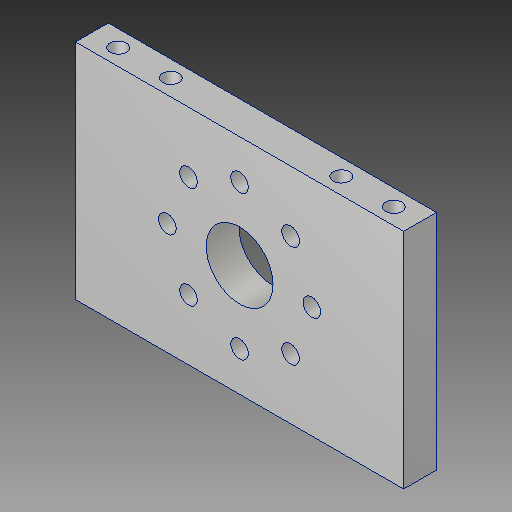
# Autodesk Inventor part: Box_Top
Saved by Autodesk Inventor 2019 (Build 230136000, 136)
## iProperties
Created: 2021-07-28
Part Number: Box_Top
Material: 알루미늄 6061
Document SubType Name: Modeling
Designer: user
Density: 2.7 g/cm^3
Appearance: 알루미늄 - 평지
Mass: 20.3803 g
Surface Area: 49.8713 cm^2
Volume: 7.54825 cm^3
Author: user
Autodesk Inventor part; units mm, degrees
ref_plane "YZ Plane" through (0, 0, 0) normal (1, 0, 0) x (0, 1, 0)
ref_plane "XZ Plane" through (0, 0, 0) normal (0, 1, 0) x (-1, 0, 0)
ref_plane "XY Plane" through (0, 0, 0) normal (0, 0, 1) x (1, 0, 0)
sketch "스케치1" plane through (0, 0, 0) normal (0, 0, 1) x (1, 0, 0)
  line L0 (-25, 17) -> (25, 17)
  line L1 (25, 17) -> (25, -17)
  line L2 (25, -17) -> (-25, -17)
  line L3 (-25, -17) -> (-25, 17)
  circle A0 centre (0, 0) radius 5.1
  line L4 (0, 0) -> (11, 0)
  line L5 (0, 0) -> (11, 0) construction
  circle A1 centre (11, 0) radius 1.35
  circle A2 centre (7.7782, 7.7782) radius 1.35
  circle A3 centre (0, 11) radius 1.35
  circle A4 centre (-7.7782, 7.7782) radius 1.35
  circle A5 centre (-11, 0) radius 1.35
  circle A6 centre (-7.7782, -7.7782) radius 1.35
  circle A7 centre (0, -11) radius 1.35
  circle A8 centre (7.7782, -7.7782) radius 1.35
  dimension "d0" = 50
  dimension "d1" = 34
  dimension "d2" = 17
  dimension "d3" = 25
  dimension "d4" = 10.2
  dimension "d5" = 11
  dimension "d6" = 0
  dimension "d7" = 2.7
  dimension "d10" = 360
  constraints: 12 end point, 9 centre point, 3 horizontal, 2 coincident, 2 parallel, 1 collinear, 1 perpendicular, 17 other
  measures "d0" distance of L1.end L2.end
  measures "d1" distance of L0.end L1.end
  measures "d2" distance from line of L0 point (0, 0)
  measures "d3" distance from line of L3 point (0, 0)
  measures "d4" diameter of A0
  measures "d5" distance of L4.start L4.end
  measures "d6" distance between parallel lines of L4 L5
  measures "d7" diameter of A1
extrude "돌출1" add sketch "스케치1" along normal blind 5
sketch "스케치2" plane through (-25, -17, 0) normal (0, -1, 0) x (1, 0, 0)
  circle A0 centre (4, 2.5) radius 1.25
  circle A1 centre (12, 2.5) radius 1.25
  circle A2 centre (38, 2.5) radius 1.25
  circle A3 centre (46, 2.5) radius 1.25
  line L0 (50, 0) -> (0, 0) projected
  line L1 (0, 0) -> (0, 5) projected
  line L2 (50, 0) -> (50, 5) projected
  point P0 (25, 0)
  dimension "d14" = 2.5
  dimension "d15" = 2.5
  dimension "d16" = 2.5
  dimension "d17" = 2.5
  dimension "d18" = 2.5
  dimension "d19" = 2.5
  dimension "d20" = 2.5
  dimension "d21" = 2.5
  dimension "d22" = 4
  dimension "d23" = 8
  dimension "d24" = 4
  dimension "d25" = 8
  constraints: 4 centre point
  measures "d14" diameter of A0
  measures "d15" diameter of A1
  measures "d16" diameter of A2
  measures "d17" diameter of A3
  measures "d18" distance from line of L0 A0.centre
  measures "d19" distance from line of L0 A1.centre
  measures "d20" distance from line of L0 A2.centre
  measures "d21" distance from line of L0 A3.centre
  measures "d22" distance from line of L1 A0.centre
  measures "d23" distance of A1.centre A0.centre
  measures "d24" distance from line of L2 A3.centre
  measures "d25" distance of A3.centre A2.centre
extrude "돌출2" cut sketch "스케치2" against normal blind 8
sketch "스케치3" plane through (-25, 17, 0) normal (0, 1, 0) x (1, 0, 0)
  circle A0 centre (38, -2.5) radius 1.25 projected
  circle A1 centre (4, -2.5) radius 1.25 projected
  circle A2 centre (12, -2.5) radius 1.25 projected
  circle A3 centre (46, -2.5) radius 1.25 projected
  line L0 (50, 0) -> (0, 0) projected
  line L1 (50, 0) -> (50, -5) projected
  line L2 (0, -5) -> (50, -5) projected
  line L3 (0, 0) -> (0, -5) projected
  point P0 (25, 0)
extrude "돌출3" cut sketch "스케치3" against normal blind 8 contours A0 | A1 | A2 | A3
equation "\"d2\" = 0.5 * d1"
equation "\"d3\" = 0.5 * d0"
equation "\"d25\" = d23"
